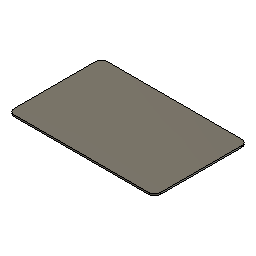
Card 3D File (Autodesk Fusion 360 design; units mm, degrees)
part number: 2026-02-12-13-33-12-488
Autodesk Fusion 360 part; units mm, degrees
(part 1 of 7)
sketch "Sketch1" plane through (0, 0, 0) normal (1, 0, 0) x (0, 0, -1)
  line L0 (-15.175, 11) -> (-93.825, 11)
  line L1 (-97, 14.175) -> (-97, 61.825)
  line L2 (-93.825, 65) -> (-15.175, 65)
  line L3 (-12, 61.825) -> (-12, 14.175)
  arc A0 (-12, 61.825) -> (-15.175, 65) centre (-15.175, 61.825) ccw
  arc A1 (-93.825, 65) -> (-97, 61.825) centre (-93.825, 61.825) ccw
  arc A2 (-97, 14.175) -> (-93.825, 11) centre (-93.825, 14.175) ccw
  arc A3 (-15.175, 11) -> (-12, 14.175) centre (-15.175, 14.175) ccw
  point P0 (-12, 11)
  point P1 (-97, 11)
  point P2 (-12, 65)
  dimension "d1" = 85
  dimension "d2" = 54
  dimension "d3" = 3.175
  dimension "d4" = 3.175
  dimension "d5" = 3.175
  constraint horizontal L0
  constraint vertical L1
  constraint horizontal L2
  constraint vertical L3
  constraint coincident P2 L2
  constraint coincident P2 L3
  constraint tangent L2 A0
  constraint tangent L3 A0
  constraint tangent L1 A1
  constraint tangent L2 A1
  constraint coincident P1 L0
  constraint coincident P1 L1
  constraint tangent L0 A2
  constraint tangent L1 A2
  constraint coincident P0 L0
  constraint coincident P0 L3
  constraint tangent L0 A3
  constraint tangent L3 A3
  constraint equal A2 A3
  measures "d1" distance of P0 P1
  measures "d2" distance of P0 P2
  measures "d3" radius of A0
  measures "d4" radius of A1
  measures "d5" radius of A2
extrude "Extrude1" add sketch "Sketch1" along normal blind 1 makes body 1
move_body "Move1" bodies 1 to x (0, -1, 0) y (1, 0, 0) z (0, 0, 1) at (-11, 11, 0)
move_body "Move2" bodies 1 to x (1, 0, 0) y (0, 1, 0) z (0, 0, 1) at (0, -10, 0)
sketch "Sketch2" plane through (0, 1, 0) normal (0, 1, 0) x (-1, 0, 0)
  arc A0 (0, 93.825) -> (-3.175, 97) centre (-3.175, 93.825) ccw
  line L0 (-3.175, 97) -> (-50.825, 97)
  arc A1 (-50.825, 97) -> (-54, 93.825) centre (-50.825, 93.825) ccw
  line L1 (-54, 93.825) -> (-54, 15.175)
  arc A2 (-54, 15.175) -> (-50.825, 12) centre (-50.825, 15.175) ccw
  line L2 (-50.825, 12) -> (-3.175, 12)
  arc A3 (-3.175, 12) -> (0, 15.175) centre (-3.175, 15.175) ccw
  line L3 (0, 15.175) -> (0, 93.825)
  line L4 (-2.9236, 18.2465) -> (-2.9236, 17.8828)
  line L5 (-2.9236, 17.8828) -> (-5.1949, 18.7001)
  line L6 (-5.1949, 18.7001) -> (-5.1949, 19.096)
  line L7 (-5.1949, 19.096) -> (-2.9236, 19.9134)
  line L8 (-2.9236, 19.9134) -> (-2.9236, 19.5496)
  line L9 (-2.9236, 19.5496) -> (-4.7824, 18.9075)
  line L10 (-4.7824, 18.9075) -> (-4.7824, 18.8898)
  line L11 (-4.7824, 18.8898) -> (-2.9236, 18.2465)
  line L12 (-3.813, 18.3075) -> (-3.813, 19.4875)
  line L13 (-3.813, 19.4875) -> (-3.5248, 19.4875)
  line L14 (-3.5248, 19.4875) -> (-3.5248, 18.3075)
  line L15 (-3.5248, 18.3075) -> (-3.813, 18.3075)
  line L16 (-2.9236, 20.2148) -> (-4.627, 20.2148)
  line L17 (-4.627, 20.2148) -> (-4.627, 20.533)
  line L18 (-4.627, 20.533) -> (-4.3498, 20.533)
  line L19 (-4.3498, 20.533) -> (-4.3498, 20.5541)
  spline S0 degree 3 poles (-4.3498, 20.5541) (-4.4437, 20.5896) (-4.5169, 20.6476) (-4.5694, 20.7282) knots 0 0 0 0 1 1 1 1
  spline S1 degree 3 poles (-4.5694, 20.7282) (-4.6226, 20.8088) (-4.6492, 20.9053) (-4.6492, 21.0177) knots 0 0 0 0 1 1 1 1
  spline S2 degree 3 poles (-4.6492, 21.0177) (-4.6492, 21.1315) (-4.6226, 21.2269) (-4.5694, 21.3038) knots 0 0 0 0 1 1 1 1
  spline S3 degree 3 poles (-4.5694, 21.3038) (-4.5161, 21.3814) (-4.4429, 21.4387) (-4.3498, 21.4757) knots 0 0 0 0 1 1 1 1
  line L20 (-4.3498, 21.4757) -> (-4.3498, 21.4935)
  spline S4 degree 3 poles (-4.3498, 21.4935) (-4.4407, 21.5341) (-4.5132, 21.5988) (-4.5672, 21.6875) knots 0 0 0 0 1 1 1 1
  spline S5 degree 3 poles (-4.5672, 21.6875) (-4.6219, 21.7763) (-4.6492, 21.882) (-4.6492, 22.0047) knots 0 0 0 0 1 1 1 1
  spline S6 degree 3 poles (-4.6492, 22.0047) (-4.6492, 22.1592) (-4.6008, 22.2853) (-4.504, 22.3829) knots 0 0 0 0 1 1 1 1
  spline S7 degree 3 poles (-4.504, 22.3829) (-4.4072, 22.4812) (-4.2612, 22.5304) (-4.066, 22.5304) knots 0 0 0 0 1 1 1 1
  line L21 (-4.066, 22.5304) -> (-2.9236, 22.5304)
  line L22 (-2.9236, 22.5304) -> (-2.9236, 22.1988)
  line L23 (-2.9236, 22.1988) -> (-4.0349, 22.1988)
  spline S8 degree 3 poles (-4.0349, 22.1988) (-4.1501, 22.1988) (-4.2337, 22.1674) (-4.2855, 22.1045) knots 0 0 0 0 1 1 1 1
  spline S9 degree 3 poles (-4.2855, 22.1045) (-4.3372, 22.0417) (-4.3631, 21.9666) (-4.3631, 21.8794) knots 0 0 0 0 1 1 1 1
  spline S10 degree 3 poles (-4.3631, 21.8794) (-4.3631, 21.7714) (-4.3299, 21.6875) (-4.2633, 21.6276) knots 0 0 0 0 1 1 1 1
  spline S11 degree 3 poles (-4.2633, 21.6276) (-4.1974, 21.5677) (-4.1128, 21.5378) (-4.0093, 21.5378) knots 0 0 0 0 1 1 1 1
  line L24 (-4.0093, 21.5378) -> (-2.9236, 21.5378)
  line L25 (-2.9236, 21.5378) -> (-2.9236, 21.2073)
  line L26 (-2.9236, 21.2073) -> (-4.056, 21.2073)
  spline S12 degree 3 poles (-4.056, 21.2073) (-4.1484, 21.2073) (-4.2226, 21.1785) (-4.2788, 21.1208) knots 0 0 0 0 1 1 1 1
  spline S13 degree 3 poles (-4.2788, 21.1208) (-4.335, 21.0632) (-4.3631, 20.9881) (-4.3631, 20.8957) knots 0 0 0 0 1 1 1 1
  spline S14 degree 3 poles (-4.3631, 20.8957) (-4.3631, 20.8328) (-4.3466, 20.7748) (-4.3132, 20.7216) knots 0 0 0 0 1 1 1 1
  spline S15 degree 3 poles (-4.3132, 20.7216) (-4.2807, 20.6691) (-4.2352, 20.6266) (-4.1768, 20.594) knots 0 0 0 0 1 1 1 1
  spline S16 degree 3 poles (-4.1768, 20.594) (-4.1184, 20.5622) (-4.0508, 20.5463) (-3.9738, 20.5463) knots 0 0 0 0 1 1 1 1
  line L27 (-3.9738, 20.5463) -> (-2.9236, 20.5463)
  line L28 (-2.9236, 20.5463) -> (-2.9236, 20.2148)
  line L29 (-2.9236, 22.9748) -> (-4.627, 22.9748)
  line L30 (-4.627, 22.9748) -> (-4.627, 23.2953)
  line L31 (-4.627, 23.2953) -> (-4.3564, 23.2953)
  line L32 (-4.3564, 23.2953) -> (-4.3564, 23.3131)
  spline S17 degree 3 poles (-4.3564, 23.3131) (-4.4482, 23.3441) (-4.5202, 23.3988) (-4.5727, 23.4772) knots 0 0 0 0 1 1 1 1
  spline S18 degree 3 poles (-4.5727, 23.4772) (-4.6259, 23.5563) (-4.6526, 23.6458) (-4.6526, 23.7456) knots 0 0 0 0 1 1 1 1
  spline S19 degree 3 poles (-4.6526, 23.7456) (-4.6526, 23.7663) (-4.6518, 23.7907) (-4.6504, 23.8188) knots 0 0 0 0 1 1 1 1
  spline S20 degree 3 poles (-4.6504, 23.8188) (-4.6489, 23.8476) (-4.647, 23.8702) (-4.6448, 23.8864) knots 0 0 0 0 1 1 1 1
  line L33 (-4.6448, 23.8864) -> (-4.3277, 23.8864)
  spline S21 degree 3 poles (-4.3277, 23.8864) (-4.3313, 23.8731) (-4.3355, 23.8495) (-4.3398, 23.8155) knots 0 0 0 0 1 1 1 1
  spline S22 degree 3 poles (-4.3398, 23.8155) (-4.345, 23.7814) (-4.3477, 23.7474) (-4.3477, 23.7134) knots 0 0 0 0 1 1 1 1
  spline S23 degree 3 poles (-4.3477, 23.7134) (-4.3477, 23.6351) (-4.3309, 23.5652) (-4.2977, 23.5038) knots 0 0 0 0 1 1 1 1
  spline S24 degree 3 poles (-4.2977, 23.5038) (-4.2652, 23.4432) (-4.2198, 23.3951) (-4.1612, 23.3596) knots 0 0 0 0 1 1 1 1
  spline S25 degree 3 poles (-4.1612, 23.3596) (-4.1036, 23.3242) (-4.0379, 23.3064) (-3.9638, 23.3064) knots 0 0 0 0 1 1 1 1
  line L34 (-3.9638, 23.3064) -> (-2.9236, 23.3064)
  line L35 (-2.9236, 23.3064) -> (-2.9236, 22.9748)
  line L36 (-2.9236, 24.1734) -> (-4.627, 24.1734)
  line L37 (-4.627, 24.1734) -> (-4.627, 24.505)
  line L38 (-4.627, 24.505) -> (-2.9236, 24.505)
  line L39 (-2.9236, 24.505) -> (-2.9236, 24.1734)
  spline S26 degree 3 poles (-4.89, 24.3408) (-4.89, 24.2832) (-4.9092, 24.2336) (-4.9476, 24.1922) knots 0 0 0 0 1 1 1 1
  spline S27 degree 3 poles (-4.9476, 24.1922) (-4.9868, 24.1516) (-5.0333, 24.1312) (-5.0873, 24.1312) knots 0 0 0 0 1 1 1 1
  spline S28 degree 3 poles (-5.0873, 24.1312) (-5.142, 24.1312) (-5.1887, 24.1516) (-5.2271, 24.1922) knots 0 0 0 0 1 1 1 1
  spline S29 degree 3 poles (-5.2271, 24.1922) (-5.2663, 24.2336) (-5.2858, 24.2832) (-5.2858, 24.3408) knots 0 0 0 0 1 1 1 1
  spline S30 degree 3 poles (-5.2858, 24.3408) (-5.2858, 24.3985) (-5.2663, 24.4477) (-5.2271, 24.4883) knots 0 0 0 0 1 1 1 1
  spline S31 degree 3 poles (-5.2271, 24.4883) (-5.1887, 24.5297) (-5.142, 24.5504) (-5.0873, 24.5504) knots 0 0 0 0 1 1 1 1
  spline S32 degree 3 poles (-5.0873, 24.5504) (-5.0333, 24.5504) (-4.9868, 24.5297) (-4.9476, 24.4883) knots 0 0 0 0 1 1 1 1
  spline S33 degree 3 poles (-4.9476, 24.4883) (-4.9092, 24.4477) (-4.89, 24.3985) (-4.89, 24.3408) knots 0 0 0 0 1 1 1 1
  line L40 (-4.627, 25.7462) -> (-4.3609, 25.7462)
  line L41 (-4.3609, 25.7462) -> (-4.3609, 24.8158)
  line L42 (-4.3609, 24.8158) -> (-4.627, 24.8158)
  line L43 (-4.627, 24.8158) -> (-4.627, 25.7462)
  line L44 (-5.0352, 25.0653) -> (-5.0352, 25.3969)
  line L45 (-5.0352, 25.3969) -> (-3.4237, 25.3969)
  spline S34 degree 3 poles (-3.4237, 25.3969) (-3.3595, 25.3969) (-3.311, 25.4065) (-3.2785, 25.4257) knots 0 0 0 0 1 1 1 1
  spline S35 degree 3 poles (-3.2785, 25.4257) (-3.2466, 25.445) (-3.2249, 25.4697) (-3.2131, 25.5) knots 0 0 0 0 1 1 1 1
  spline S36 degree 3 poles (-3.2131, 25.5) (-3.202, 25.5311) (-3.1964, 25.5647) (-3.1964, 25.601) knots 0 0 0 0 1 1 1 1
  spline S37 degree 3 poles (-3.1964, 25.601) (-3.1964, 25.6276) (-3.1982, 25.6509) (-3.202, 25.6708) knots 0 0 0 0 1 1 1 1
  spline S38 degree 3 poles (-3.202, 25.6708) (-3.2057, 25.6908) (-3.2087, 25.7063) (-3.2109, 25.7174) knots 0 0 0 0 1 1 1 1
  line L46 (-3.2109, 25.7174) -> (-2.937, 25.7773)
  spline S39 degree 3 poles (-2.937, 25.7773) (-2.9295, 25.7581) (-2.9222, 25.7307) (-2.9147, 25.6952) knots 0 0 0 0 1 1 1 1
  spline S40 degree 3 poles (-2.9147, 25.6952) (-2.9066, 25.6597) (-2.9022, 25.6154) (-2.9014, 25.5621) knots 0 0 0 0 1 1 1 1
  spline S41 degree 3 poles (-2.9014, 25.5621) (-2.9, 25.4749) (-2.9155, 25.3936) (-2.9481, 25.3182) knots 0 0 0 0 1 1 1 1
  spline S42 degree 3 poles (-2.9481, 25.3182) (-2.9806, 25.2427) (-3.0309, 25.1818) (-3.0988, 25.1352) knots 0 0 0 0 1 1 1 1
  spline S43 degree 3 poles (-3.0988, 25.1352) (-3.1669, 25.0886) (-3.2523, 25.0653) (-3.355, 25.0653) knots 0 0 0 0 1 1 1 1
  line L47 (-3.355, 25.0653) -> (-5.0352, 25.0653)
  spline S44 degree 3 poles (-12.1187, 79.4371) (-12.12, 79.1129) (-12.1998, 78.8339) (-12.3581, 78.6001) knots 0 0 0 0 1 1 1 1
  spline S45 degree 3 poles (-12.3581, 78.6001) (-12.5164, 78.3675) (-12.7458, 78.1884) (-13.0463, 78.0628) knots 0 0 0 0 1 1 1 1
  spline S46 degree 3 poles (-13.0463, 78.0628) (-13.3467, 77.9384) (-13.708, 77.8767) (-14.1302, 77.8779) knots 0 0 0 0 1 1 1 1
  spline S47 degree 3 poles (-14.1302, 77.8779) (-14.5514, 77.8779) (-14.9102, 77.9402) (-15.2069, 78.0647) knots 0 0 0 0 1 1 1 1
  spline S48 degree 3 poles (-15.2069, 78.0647) (-15.5034, 78.1904) (-15.7291, 78.3695) (-15.8836, 78.602) knots 0 0 0 0 1 1 1 1
  spline S49 degree 3 poles (-15.8836, 78.602) (-16.0395, 78.8358) (-16.1174, 79.1142) (-16.1174, 79.4371) knots 0 0 0 0 1 1 1 1
  spline S50 degree 3 poles (-16.1174, 79.4371) (-16.1174, 79.7602) (-16.0395, 80.0379) (-15.8836, 80.2704) knots 0 0 0 0 1 1 1 1
  spline S51 degree 3 poles (-15.8836, 80.2704) (-15.7278, 80.5042) (-15.5015, 80.6839) (-15.205, 80.8096) knots 0 0 0 0 1 1 1 1
  spline S52 degree 3 poles (-15.205, 80.8096) (-14.9096, 80.9353) (-14.5514, 80.9976) (-14.1302, 80.9962) knots 0 0 0 0 1 1 1 1
  spline S53 degree 3 poles (-14.1302, 80.9962) (-13.7068, 80.9962) (-13.3448, 80.9335) (-13.0444, 80.8078) knots 0 0 0 0 1 1 1 1
  spline S54 degree 3 poles (-13.0444, 80.8078) (-12.744, 80.6833) (-12.5146, 80.5048) (-12.3562, 80.2723) knots 0 0 0 0 1 1 1 1
  spline S55 degree 3 poles (-12.3562, 80.2723) (-12.1979, 80.0398) (-12.1187, 79.7614) (-12.1187, 79.4371) knots 0 0 0 0 1 1 1 1
  spline S56 degree 3 poles (-12.7955, 79.4371) (-12.7955, 79.6583) (-12.9068, 79.8349) (-13.1292, 79.9669) knots 0 0 0 0 1 1 1 1
  spline S57 degree 3 poles (-13.1292, 79.9669) (-13.3517, 80.0988) (-13.6854, 80.1643) (-14.1302, 80.163) knots 0 0 0 0 1 1 1 1
  spline S58 degree 3 poles (-14.1302, 80.163) (-14.4232, 80.163) (-14.6671, 80.1329) (-14.8618, 80.0725) knots 0 0 0 0 1 1 1 1
  spline S59 degree 3 poles (-14.8618, 80.0725) (-15.0567, 80.0134) (-15.2031, 79.9293) (-15.301, 79.8198) knots 0 0 0 0 1 1 1 1
  spline S60 degree 3 poles (-15.301, 79.8198) (-15.3991, 79.7117) (-15.4481, 79.5842) (-15.4481, 79.4371) knots 0 0 0 0 1 1 1 1
  spline S61 degree 3 poles (-15.4481, 79.4371) (-15.4481, 79.2172) (-15.3382, 79.0412) (-15.1182, 78.9093) knots 0 0 0 0 1 1 1 1
  spline S62 degree 3 poles (-15.1182, 78.9093) (-14.8983, 78.7773) (-14.569, 78.7107) (-14.1302, 78.7094) knots 0 0 0 0 1 1 1 1
  spline S63 degree 3 poles (-14.1302, 78.7094) (-13.8337, 78.7094) (-13.5861, 78.7389) (-13.3874, 78.798) knots 0 0 0 0 1 1 1 1
  spline S64 degree 3 poles (-13.3874, 78.798) (-13.1902, 78.8584) (-13.0419, 78.9432) (-12.9426, 79.0525) knots 0 0 0 0 1 1 1 1
  spline S65 degree 3 poles (-12.9426, 79.0525) (-12.8445, 79.1619) (-12.7955, 79.2901) (-12.7955, 79.4371) knots 0 0 0 0 1 1 1 1
  line L48 (-12.2035, 81.5783) -> (-12.7917, 81.5783)
  line L49 (-12.7917, 81.5783) -> (-14.0643, 82.9528)
  spline S66 degree 3 poles (-14.0643, 82.9528) (-14.1774, 83.0697) (-14.2792, 83.1678) (-14.3698, 83.247) knots 0 0 0 0 1 1 1 1
  spline S67 degree 3 poles (-14.3698, 83.247) (-14.4602, 83.3274) (-14.5489, 83.3883) (-14.6355, 83.4298) knots 0 0 0 0 1 1 1 1
  spline S68 degree 3 poles (-14.6355, 83.4298) (-14.7236, 83.4712) (-14.8184, 83.492) (-14.9202, 83.492) knots 0 0 0 0 1 1 1 1
  spline S69 degree 3 poles (-14.9202, 83.492) (-15.0334, 83.492) (-15.1308, 83.4662) (-15.2125, 83.4147) knots 0 0 0 0 1 1 1 1
  spline S70 degree 3 poles (-15.2125, 83.4147) (-15.2954, 83.3631) (-15.359, 83.2927) (-15.4029, 83.2036) knots 0 0 0 0 1 1 1 1
  spline S71 degree 3 poles (-15.4029, 83.2036) (-15.4481, 83.1142) (-15.4708, 83.0131) (-15.4708, 82.9) knots 0 0 0 0 1 1 1 1
  spline S72 degree 3 poles (-15.4708, 82.9) (-15.4708, 82.7818) (-15.4469, 82.6787) (-15.3991, 82.5908) knots 0 0 0 0 1 1 1 1
  spline S73 degree 3 poles (-15.3991, 82.5908) (-15.3513, 82.5028) (-15.2829, 82.435) (-15.1936, 82.3872) knots 0 0 0 0 1 1 1 1
  spline S74 degree 3 poles (-15.1936, 82.3872) (-15.1045, 82.3394) (-14.9981, 82.3155) (-14.8751, 82.3155) knots 0 0 0 0 1 1 1 1
  line L50 (-14.8751, 82.3155) -> (-14.8751, 81.5407)
  spline S75 degree 3 poles (-14.8751, 81.5407) (-15.1277, 81.5407) (-15.347, 81.5979) (-15.5329, 81.7123) knots 0 0 0 0 1 1 1 1
  spline S76 degree 3 poles (-15.5329, 81.7123) (-15.7191, 81.8266) (-15.8629, 81.9868) (-15.9647, 82.193) knots 0 0 0 0 1 1 1 1
  spline S77 degree 3 poles (-15.9647, 82.193) (-16.0665, 82.3991) (-16.1174, 82.6367) (-16.1174, 82.9056) knots 0 0 0 0 1 1 1 1
  spline S78 degree 3 poles (-16.1174, 82.9056) (-16.1174, 83.1822) (-16.0684, 83.4229) (-15.9705, 83.6278) knots 0 0 0 0 1 1 1 1
  spline S79 degree 3 poles (-15.9705, 83.6278) (-15.8736, 83.8339) (-15.7392, 83.9941) (-15.567, 84.1084) knots 0 0 0 0 1 1 1 1
  spline S80 degree 3 poles (-15.567, 84.1084) (-15.3947, 84.2229) (-15.1974, 84.28) (-14.975, 84.28) knots 0 0 0 0 1 1 1 1
  spline S81 degree 3 poles (-14.975, 84.28) (-14.8292, 84.28) (-14.6852, 84.2512) (-14.5433, 84.1934) knots 0 0 0 0 1 1 1 1
  spline S82 degree 3 poles (-14.5433, 84.1934) (-14.4012, 84.1367) (-14.2434, 84.0357) (-14.07, 83.8898) knots 0 0 0 0 1 1 1 1
  spline S83 degree 3 poles (-14.07, 83.8898) (-13.8977, 83.744) (-13.691, 83.5385) (-13.4497, 83.2733) knots 0 0 0 0 1 1 1 1
  line L51 (-13.4497, 83.2733) -> (-12.8973, 82.7097)
  line L52 (-12.8973, 82.7097) -> (-12.8709, 82.7097)
  line L53 (-12.8709, 82.7097) -> (-12.8709, 84.3309)
  line L54 (-12.8709, 84.3309) -> (-12.2035, 84.3309)
  line L55 (-12.2035, 84.3309) -> (-12.2035, 81.5783)
  line L56 (-16.2456, 86.6117) -> (-11.6228, 85.3675)
  line L57 (-11.6228, 85.3675) -> (-11.6228, 84.6756)
  line L58 (-11.6228, 84.6756) -> (-16.2456, 85.9198)
  line L59 (-16.2456, 85.9198) -> (-16.2456, 86.6117)
  spline S84 degree 3 poles (-12.1507, 88.4183) (-12.1507, 88.1368) (-12.1991, 87.886) (-12.296, 87.6661) knots 0 0 0 0 1 1 1 1
  spline S85 degree 3 poles (-12.296, 87.6661) (-12.3939, 87.4474) (-12.5285, 87.2745) (-12.6993, 87.1476) knots 0 0 0 0 1 1 1 1
  spline S86 degree 3 poles (-12.6993, 87.1476) (-12.8715, 87.022) (-13.0701, 86.9572) (-13.2952, 86.9535) knots 0 0 0 0 1 1 1 1
  line L60 (-13.2952, 86.9535) -> (-13.2952, 87.7754)
  spline S87 degree 3 poles (-13.2952, 87.7754) (-13.2008, 87.7804) (-13.1179, 87.8112) (-13.0463, 87.8679) knots 0 0 0 0 1 1 1 1
  spline S88 degree 3 poles (-13.0463, 87.8679) (-12.9758, 87.9257) (-12.9212, 88.0023) (-12.8823, 88.0979) knots 0 0 0 0 1 1 1 1
  spline S89 degree 3 poles (-12.8823, 88.0979) (-12.8433, 88.1933) (-12.8237, 88.3009) (-12.8237, 88.4202) knots 0 0 0 0 1 1 1 1
  spline S90 degree 3 poles (-12.8237, 88.4202) (-12.8237, 88.5446) (-12.8458, 88.6546) (-12.8898, 88.7501) knots 0 0 0 0 1 1 1 1
  spline S91 degree 3 poles (-12.8898, 88.7501) (-12.9338, 88.8457) (-12.9947, 88.9205) (-13.0726, 88.9745) knots 0 0 0 0 1 1 1 1
  spline S92 degree 3 poles (-13.0726, 88.9745) (-13.1506, 89.0285) (-13.2405, 89.0556) (-13.3423, 89.0556) knots 0 0 0 0 1 1 1 1
  spline S93 degree 3 poles (-13.3423, 89.0556) (-13.4454, 89.0556) (-13.5364, 89.0267) (-13.6156, 88.9689) knots 0 0 0 0 1 1 1 1
  spline S94 degree 3 poles (-13.6156, 88.9689) (-13.696, 88.9124) (-13.7589, 88.8305) (-13.8042, 88.7237) knots 0 0 0 0 1 1 1 1
  spline S95 degree 3 poles (-13.8042, 88.7237) (-13.8493, 88.6182) (-13.872, 88.4925) (-13.872, 88.3466) knots 0 0 0 0 1 1 1 1
  line L61 (-13.872, 88.3466) -> (-13.872, 87.9866)
  line L62 (-13.872, 87.9866) -> (-14.4716, 87.9866)
  line L63 (-14.4716, 87.9866) -> (-14.4716, 88.3466)
  spline S96 degree 3 poles (-14.4716, 88.3466) (-14.4716, 88.4698) (-14.493, 88.5787) (-14.5356, 88.6728) knots 0 0 0 0 1 1 1 1
  spline S97 degree 3 poles (-14.5356, 88.6728) (-14.5784, 88.7684) (-14.6374, 88.8426) (-14.7128, 88.8953) knots 0 0 0 0 1 1 1 1
  spline S98 degree 3 poles (-14.7128, 88.8953) (-14.7895, 88.9481) (-14.8788, 88.9745) (-14.9806, 88.9745) knots 0 0 0 0 1 1 1 1
  spline S99 degree 3 poles (-14.9806, 88.9745) (-15.0774, 88.9745) (-15.1622, 88.9512) (-15.2352, 88.9047) knots 0 0 0 0 1 1 1 1
  spline S100 degree 3 poles (-15.2352, 88.9047) (-15.3093, 88.8596) (-15.3671, 88.7954) (-15.4086, 88.7125) knots 0 0 0 0 1 1 1 1
  spline S101 degree 3 poles (-15.4086, 88.7125) (-15.45, 88.6308) (-15.4708, 88.5353) (-15.4708, 88.426) knots 0 0 0 0 1 1 1 1
  spline S102 degree 3 poles (-15.4708, 88.426) (-15.4708, 88.3152) (-15.4506, 88.2141) (-15.4105, 88.1224) knots 0 0 0 0 1 1 1 1
  spline S103 degree 3 poles (-15.4105, 88.1224) (-15.3715, 88.0306) (-15.3156, 87.957) (-15.2426, 87.9018) knots 0 0 0 0 1 1 1 1
  spline S104 degree 3 poles (-15.2426, 87.9018) (-15.1697, 87.8465) (-15.0843, 87.817) (-14.9862, 87.8132) knots 0 0 0 0 1 1 1 1
  line L64 (-14.9862, 87.8132) -> (-14.9862, 87.0308)
  spline S105 degree 3 poles (-14.9862, 87.0308) (-15.2088, 87.0345) (-15.4047, 87.0981) (-15.5745, 87.2211) knots 0 0 0 0 1 1 1 1
  spline S106 degree 3 poles (-15.5745, 87.2211) (-15.7442, 87.3443) (-15.8768, 87.5103) (-15.9723, 87.7189) knots 0 0 0 0 1 1 1 1
  spline S107 degree 3 poles (-15.9723, 87.7189) (-16.069, 87.9288) (-16.1174, 88.1657) (-16.1174, 88.4297) knots 0 0 0 0 1 1 1 1
  spline S108 degree 3 poles (-16.1174, 88.4297) (-16.1174, 88.6961) (-16.069, 88.9292) (-15.9723, 89.1291) knots 0 0 0 0 1 1 1 1
  spline S109 degree 3 poles (-15.9723, 89.1291) (-15.8755, 89.329) (-15.7448, 89.4842) (-15.5801, 89.5947) knots 0 0 0 0 1 1 1 1
  spline S110 degree 3 poles (-15.5801, 89.5947) (-15.4168, 89.7067) (-15.2333, 89.762) (-15.0297, 89.7607) knots 0 0 0 0 1 1 1 1
  spline S111 degree 3 poles (-15.0297, 89.7607) (-14.8134, 89.762) (-14.633, 89.6947) (-14.4886, 89.559) knots 0 0 0 0 1 1 1 1
  spline S112 degree 3 poles (-14.4886, 89.559) (-14.344, 89.4245) (-14.2522, 89.2492) (-14.2133, 89.0329) knots 0 0 0 0 1 1 1 1
  line L65 (-14.2133, 89.0329) -> (-14.1832, 89.0329)
  spline S113 degree 3 poles (-14.1832, 89.0329) (-14.1466, 89.317) (-14.048, 89.5332) (-13.8871, 89.6816) knots 0 0 0 0 1 1 1 1
  spline S114 degree 3 poles (-13.8871, 89.6816) (-13.7275, 89.8312) (-13.5277, 89.9052) (-13.2875, 89.9039) knots 0 0 0 0 1 1 1 1
  spline S115 degree 3 poles (-13.2875, 89.9039) (-13.0676, 89.9052) (-12.8722, 89.8418) (-12.7013, 89.7136) knots 0 0 0 0 1 1 1 1
  spline S116 degree 3 poles (-12.7013, 89.7136) (-12.5303, 89.5866) (-12.3959, 89.4113) (-12.2978, 89.1875) knots 0 0 0 0 1 1 1 1
  spline S117 degree 3 poles (-12.2978, 89.1875) (-12.1998, 88.9639) (-12.1507, 88.7075) (-12.1507, 88.4183) knots 0 0 0 0 1 1 1 1
  spline S118 degree 3 poles (-12.1187, 92.0047) (-12.12, 91.6804) (-12.1998, 91.4014) (-12.3581, 91.1676) knots 0 0 0 0 1 1 1 1
  spline S119 degree 3 poles (-12.3581, 91.1676) (-12.5164, 90.9351) (-12.7458, 90.756) (-13.0463, 90.6303) knots 0 0 0 0 1 1 1 1
  spline S120 degree 3 poles (-13.0463, 90.6303) (-13.3467, 90.5059) (-13.708, 90.4443) (-14.1302, 90.4456) knots 0 0 0 0 1 1 1 1
  spline S121 degree 3 poles (-14.1302, 90.4456) (-14.5514, 90.4456) (-14.9102, 90.5077) (-15.2069, 90.6322) knots 0 0 0 0 1 1 1 1
  spline S122 degree 3 poles (-15.2069, 90.6322) (-15.5034, 90.7579) (-15.7291, 90.937) (-15.8836, 91.1695) knots 0 0 0 0 1 1 1 1
  spline S123 degree 3 poles (-15.8836, 91.1695) (-16.0395, 91.4033) (-16.1174, 91.6817) (-16.1174, 92.0047) knots 0 0 0 0 1 1 1 1
  spline S124 degree 3 poles (-16.1174, 92.0047) (-16.1174, 92.3277) (-16.0395, 92.6054) (-15.8836, 92.8379) knots 0 0 0 0 1 1 1 1
  spline S125 degree 3 poles (-15.8836, 92.8379) (-15.7278, 93.0719) (-15.5015, 93.2516) (-15.205, 93.3773) knots 0 0 0 0 1 1 1 1
  spline S126 degree 3 poles (-15.205, 93.3773) (-14.9096, 93.5028) (-14.5514, 93.5651) (-14.1302, 93.5639) knots 0 0 0 0 1 1 1 1
  spline S127 degree 3 poles (-14.1302, 93.5639) (-13.7068, 93.5639) (-13.3448, 93.501) (-13.0444, 93.3753) knots 0 0 0 0 1 1 1 1
  spline S128 degree 3 poles (-13.0444, 93.3753) (-12.744, 93.251) (-12.5146, 93.0725) (-12.3562, 92.8398) knots 0 0 0 0 1 1 1 1
  spline S129 degree 3 poles (-12.3562, 92.8398) (-12.1979, 92.6073) (-12.1187, 92.3289) (-12.1187, 92.0047) knots 0 0 0 0 1 1 1 1
  spline S130 degree 3 poles (-12.7955, 92.0047) (-12.7955, 92.2258) (-12.9068, 92.4024) (-13.1292, 92.5346) knots 0 0 0 0 1 1 1 1
  spline S131 degree 3 poles (-13.1292, 92.5346) (-13.3517, 92.6665) (-13.6854, 92.7318) (-14.1302, 92.7305) knots 0 0 0 0 1 1 1 1
  spline S132 degree 3 poles (-14.1302, 92.7305) (-14.4232, 92.7305) (-14.6671, 92.7004) (-14.8618, 92.6401) knots 0 0 0 0 1 1 1 1
  spline S133 degree 3 poles (-14.8618, 92.6401) (-15.0567, 92.5809) (-15.2031, 92.4968) (-15.301, 92.3875) knots 0 0 0 0 1 1 1 1
  spline S134 degree 3 poles (-15.301, 92.3875) (-15.3991, 92.2794) (-15.4481, 92.1518) (-15.4481, 92.0047) knots 0 0 0 0 1 1 1 1
  spline S135 degree 3 poles (-15.4481, 92.0047) (-15.4481, 91.7847) (-15.3382, 91.6087) (-15.1182, 91.4768) knots 0 0 0 0 1 1 1 1
  spline S136 degree 3 poles (-15.1182, 91.4768) (-14.8983, 91.3449) (-14.569, 91.2782) (-14.1302, 91.2769) knots 0 0 0 0 1 1 1 1
  spline S137 degree 3 poles (-14.1302, 91.2769) (-13.8337, 91.2769) (-13.5861, 91.3064) (-13.3874, 91.3656) knots 0 0 0 0 1 1 1 1
  spline S138 degree 3 poles (-13.3874, 91.3656) (-13.1902, 91.4259) (-13.0419, 91.5107) (-12.9426, 91.6201) knots 0 0 0 0 1 1 1 1
  spline S139 degree 3 poles (-12.9426, 91.6201) (-12.8445, 91.7294) (-12.7955, 91.8576) (-12.7955, 92.0047) knots 0 0 0 0 1 1 1 1
  spline S140 degree 3 poles (-48.5277, 92.7546) (-48.5876, 92.8726) (-48.5469, 92.9888) (-48.4658, 93.03) knots 0 0 0 0 1 1 1 1
  line L66 (-48.4658, 93.03) -> (-48.4623, 93.0318)
  line L67 (-48.4623, 93.0318) -> (-48.4588, 93.0338)
  spline S141 degree 3 poles (-48.4588, 93.0338) (-47.5901, 93.5364) (-46.5968, 93.8317) (-45.5192, 93.8373) knots 0 0 0 0 1 1 1 1
  spline S142 degree 3 poles (-45.5192, 93.8373) (-44.4427, 93.8431) (-43.4474, 93.5591) (-42.574, 93.0667) knots 0 0 0 0 1 1 1 1
  spline S143 degree 3 poles (-42.574, 93.0667) (-42.4748, 93.0041) (-42.447, 92.8992) (-42.4965, 92.7928) knots 0 0 0 0 1 1 1 1
  spline S144 degree 3 poles (-42.4965, 92.7928) (-42.5596, 92.696) (-42.6642, 92.6696) (-42.7699, 92.7198) knots 0 0 0 0 1 1 1 1
  spline S145 degree 3 poles (-42.7699, 92.7198) (-43.5795, 93.1942) (-44.5173, 93.4496) (-45.5171, 93.4443) knots 0 0 0 0 1 1 1 1
  spline S146 degree 3 poles (-45.5171, 93.4443) (-46.5195, 93.4389) (-47.4538, 93.151) (-48.2554, 92.6912) knots 0 0 0 0 1 1 1 1
  spline S147 degree 3 poles (-48.2554, 92.6912) (-48.3724, 92.6336) (-48.487, 92.6742) (-48.5277, 92.7546) knots 0 0 0 0 1 1 1 1
  spline S148 degree 3 poles (-47.8872, 91.5327) (-47.9426, 91.6486) (-47.902, 91.7616) (-47.8223, 91.8021) knots 0 0 0 0 1 1 1 1
  line L68 (-47.8223, 91.8021) -> (-47.8171, 91.8047)
  line L69 (-47.8171, 91.8047) -> (-47.8121, 91.8076)
  spline S149 degree 3 poles (-47.8121, 91.8076) (-47.1359, 92.2224) (-46.356, 92.453) (-45.5119, 92.4575) knots 0 0 0 0 1 1 1 1
  spline S150 degree 3 poles (-45.5119, 92.4575) (-44.6681, 92.4619) (-43.8861, 92.24) (-43.2058, 91.8328) knots 0 0 0 0 1 1 1 1
  spline S151 degree 3 poles (-43.2058, 91.8328) (-43.1054, 91.7703) (-43.0771, 91.6649) (-43.1268, 91.5581) knots 0 0 0 0 1 1 1 1
  spline S152 degree 3 poles (-43.1268, 91.5581) (-43.1902, 91.461) (-43.2952, 91.4349) (-43.4012, 91.4856) knots 0 0 0 0 1 1 1 1
  spline S153 degree 3 poles (-43.4012, 91.4856) (-44.0162, 91.8318) (-44.7408, 92.0473) (-45.5097, 92.0431) knots 0 0 0 0 1 1 1 1
  spline S154 degree 3 poles (-45.5097, 92.0431) (-46.2751, 92.039) (-46.9986, 91.8388) (-47.6135, 91.4624) knots 0 0 0 0 1 1 1 1
  spline S155 degree 3 poles (-47.6135, 91.4624) (-47.7185, 91.4115) (-47.8231, 91.4367) (-47.8872, 91.5327) knots 0 0 0 0 1 1 1 1
  spline S156 degree 3 poles (-47.2523, 90.2965) (-47.3004, 90.363) (-47.2833, 90.4878) (-47.1841, 90.5618) knots 0 0 0 0 1 1 1 1
  spline S157 degree 3 poles (-47.1841, 90.5618) (-46.6984, 90.868) (-46.1114, 91.0529) (-45.5044, 91.056) knots 0 0 0 0 1 1 1 1
  spline S158 degree 3 poles (-45.5044, 91.056) (-44.8767, 91.0595) (-44.3087, 90.8809) (-43.8196, 90.5797) knots 0 0 0 0 1 1 1 1
  spline S159 degree 3 poles (-43.8196, 90.5797) (-43.7237, 90.5101) (-43.6969, 90.4034) (-43.7512, 90.3115) knots 0 0 0 0 1 1 1 1
  spline S160 degree 3 poles (-43.7512, 90.3115) (-43.8242, 90.2118) (-43.9486, 90.1936) (-44.0156, 90.2407) knots 0 0 0 0 1 1 1 1
  line L70 (-44.0156, 90.2407) -> (-44.0189, 90.2433)
  line L71 (-44.0189, 90.2433) -> (-44.0224, 90.2456)
  spline S161 degree 3 poles (-44.0224, 90.2456) (-44.4497, 90.5122) (-44.9652, 90.6662) (-45.5023, 90.6633) knots 0 0 0 0 1 1 1 1
  spline S162 degree 3 poles (-45.5023, 90.6633) (-46.0393, 90.6604) (-46.5531, 90.5011) (-46.9775, 90.23) knots 0 0 0 0 1 1 1 1
  spline S163 degree 3 poles (-46.9775, 90.23) (-47.0706, 90.1713) (-47.1808, 90.1977) (-47.2523, 90.2965) knots 0 0 0 0 1 1 1 1
  spline S164 degree 3 poles (-46.6301, 89.0896) (-46.6974, 89.1827) (-46.6763, 89.3029) (-46.6011, 89.3572) knots 0 0 0 0 1 1 1 1
  line L72 (-46.6011, 89.3572) -> (-46.5999, 89.3581)
  line L73 (-46.5999, 89.3581) -> (-46.5985, 89.3593)
  spline S165 degree 3 poles (-46.5985, 89.3593) (-46.4398, 89.4795) (-46.2634, 89.5782) (-46.0905, 89.6372) knots 0 0 0 0 1 1 1 1
  spline S166 degree 3 poles (-46.0905, 89.6372) (-45.8871, 89.6992) (-45.6903, 89.7387) (-45.4974, 89.7398) knots 0 0 0 0 1 1 1 1
  spline S167 degree 3 poles (-45.4974, 89.7398) (-45.2944, 89.741) (-45.1023, 89.7214) (-44.9132, 89.6469) knots 0 0 0 0 1 1 1 1
  spline S168 degree 3 poles (-44.9132, 89.6469) (-44.7072, 89.5658) (-44.5492, 89.4873) (-44.3923, 89.371) knots 0 0 0 0 1 1 1 1
  line L74 (-44.3923, 89.371) -> (-44.3911, 89.3698)
  line L75 (-44.3911, 89.3698) -> (-44.3897, 89.3689)
  spline S169 degree 3 poles (-44.3897, 89.3689) (-44.3139, 89.3154) (-44.2915, 89.1955) (-44.3578, 89.1016) knots 0 0 0 0 1 1 1 1
  spline S170 degree 3 poles (-44.3578, 89.1016) (-44.4108, 89.0267) (-44.5289, 89.004) (-44.6223, 89.0679) knots 0 0 0 0 1 1 1 1
  spline S171 degree 3 poles (-44.6223, 89.0679) (-44.7439, 89.1633) (-44.8861, 89.2326) (-45.0251, 89.2781) knots 0 0 0 0 1 1 1 1
  spline S172 degree 3 poles (-45.0251, 89.2781) (-45.1697, 89.3254) (-45.3341, 89.3476) (-45.4953, 89.3466) knots 0 0 0 0 1 1 1 1
  spline S173 degree 3 poles (-45.4953, 89.3466) (-45.6565, 89.3458) (-45.8207, 89.3219) (-45.9649, 89.2731) knots 0 0 0 0 1 1 1 1
  spline S174 degree 3 poles (-45.9649, 89.2731) (-46.1033, 89.2261) (-46.2447, 89.1553) (-46.3652, 89.0587) knots 0 0 0 0 1 1 1 1
  spline S175 degree 3 poles (-46.3652, 89.0587) (-46.4579, 88.9937) (-46.5763, 89.0151) (-46.6301, 89.0896) knots 0 0 0 0 1 1 1 1
  line L76 (-9.9923, 17.8051) -> (-9.9923, 94.3182)
  spline S176 degree 3 poles (-12.1507, 19.233) (-12.1507, 18.9515) (-12.1991, 18.7007) (-12.296, 18.4808) knots 0 0 0 0 1 1 1 1
  spline S177 degree 3 poles (-12.296, 18.4808) (-12.3939, 18.2621) (-12.5285, 18.0892) (-12.6993, 17.9623) knots 0 0 0 0 1 1 1 1
  spline S178 degree 3 poles (-12.6993, 17.9623) (-12.8715, 17.8366) (-13.0701, 17.7719) (-13.2952, 17.7681) knots 0 0 0 0 1 1 1 1
  line L77 (-13.2952, 17.7681) -> (-13.2952, 18.5901)
  spline S179 degree 3 poles (-13.2952, 18.5901) (-13.2008, 18.5951) (-13.1179, 18.6259) (-13.0463, 18.6825) knots 0 0 0 0 1 1 1 1
  spline S180 degree 3 poles (-13.0463, 18.6825) (-12.9758, 18.7403) (-12.9212, 18.817) (-12.8823, 18.9125) knots 0 0 0 0 1 1 1 1
  spline S181 degree 3 poles (-12.8823, 18.9125) (-12.8433, 19.008) (-12.8237, 19.1155) (-12.8237, 19.2349) knots 0 0 0 0 1 1 1 1
  spline S182 degree 3 poles (-12.8237, 19.2349) (-12.8237, 19.3593) (-12.8458, 19.4693) (-12.8898, 19.5648) knots 0 0 0 0 1 1 1 1
  spline S183 degree 3 poles (-12.8898, 19.5648) (-12.9338, 19.6603) (-12.9947, 19.7351) (-13.0726, 19.7892) knots 0 0 0 0 1 1 1 1
  spline S184 degree 3 poles (-13.0726, 19.7892) (-13.1506, 19.8432) (-13.2405, 19.8702) (-13.3423, 19.8702) knots 0 0 0 0 1 1 1 1
  spline S185 degree 3 poles (-13.3423, 19.8702) (-13.4454, 19.8702) (-13.5364, 19.8413) (-13.6156, 19.7835) knots 0 0 0 0 1 1 1 1
  spline S186 degree 3 poles (-13.6156, 19.7835) (-13.696, 19.727) (-13.7589, 19.6453) (-13.8042, 19.5384) knots 0 0 0 0 1 1 1 1
  spline S187 degree 3 poles (-13.8042, 19.5384) (-13.8493, 19.4328) (-13.872, 19.3072) (-13.872, 19.1614) knots 0 0 0 0 1 1 1 1
  line L78 (-13.872, 19.1614) -> (-13.872, 18.8013)
  line L79 (-13.872, 18.8013) -> (-14.4716, 18.8013)
  line L80 (-14.4716, 18.8013) -> (-14.4716, 19.1614)
  spline S188 degree 3 poles (-14.4716, 19.1614) (-14.4716, 19.2845) (-14.493, 19.3933) (-14.5356, 19.4875) knots 0 0 0 0 1 1 1 1
  spline S189 degree 3 poles (-14.5356, 19.4875) (-14.5784, 19.583) (-14.6374, 19.6572) (-14.7128, 19.71) knots 0 0 0 0 1 1 1 1
  spline S190 degree 3 poles (-14.7128, 19.71) (-14.7895, 19.7628) (-14.8788, 19.7892) (-14.9806, 19.7892) knots 0 0 0 0 1 1 1 1
  spline S191 degree 3 poles (-14.9806, 19.7892) (-15.0774, 19.7892) (-15.1622, 19.7659) (-15.2352, 19.7194) knots 0 0 0 0 1 1 1 1
  spline S192 degree 3 poles (-15.2352, 19.7194) (-15.3093, 19.6742) (-15.3671, 19.6101) (-15.4086, 19.5271) knots 0 0 0 0 1 1 1 1
  spline S193 degree 3 poles (-15.4086, 19.5271) (-15.45, 19.4454) (-15.4708, 19.3499) (-15.4708, 19.2405) knots 0 0 0 0 1 1 1 1
  spline S194 degree 3 poles (-15.4708, 19.2405) (-15.4708, 19.1299) (-15.4506, 19.0288) (-15.4105, 18.937) knots 0 0 0 0 1 1 1 1
  spline S195 degree 3 poles (-15.4105, 18.937) (-15.3715, 18.8453) (-15.3156, 18.7717) (-15.2426, 18.7164) knots 0 0 0 0 1 1 1 1
  spline S196 degree 3 poles (-15.2426, 18.7164) (-15.1697, 18.6611) (-15.0843, 18.6316) (-14.9862, 18.6278) knots 0 0 0 0 1 1 1 1
  line L81 (-14.9862, 18.6278) -> (-14.9862, 17.8454)
  spline S197 degree 3 poles (-14.9862, 17.8454) (-15.2088, 17.8492) (-15.4047, 17.9126) (-15.5745, 18.0358) knots 0 0 0 0 1 1 1 1
  spline S198 degree 3 poles (-15.5745, 18.0358) (-15.7442, 18.159) (-15.8768, 18.3249) (-15.9723, 18.5335) knots 0 0 0 0 1 1 1 1
  spline S199 degree 3 poles (-15.9723, 18.5335) (-16.069, 18.7434) (-16.1174, 18.9804) (-16.1174, 19.2443) knots 0 0 0 0 1 1 1 1
  spline S200 degree 3 poles (-16.1174, 19.2443) (-16.1174, 19.5108) (-16.069, 19.7439) (-15.9723, 19.9438) knots 0 0 0 0 1 1 1 1
  spline S201 degree 3 poles (-15.9723, 19.9438) (-15.8755, 20.1436) (-15.7448, 20.2988) (-15.5801, 20.4094) knots 0 0 0 0 1 1 1 1
  spline S202 degree 3 poles (-15.5801, 20.4094) (-15.4168, 20.5213) (-15.2333, 20.5766) (-15.0297, 20.5754) knots 0 0 0 0 1 1 1 1
  spline S203 degree 3 poles (-15.0297, 20.5754) (-14.8134, 20.5766) (-14.633, 20.5094) (-14.4886, 20.3736) knots 0 0 0 0 1 1 1 1
  spline S204 degree 3 poles (-14.4886, 20.3736) (-14.344, 20.2391) (-14.2522, 20.0638) (-14.2133, 19.8476) knots 0 0 0 0 1 1 1 1
  line L82 (-14.2133, 19.8476) -> (-14.1832, 19.8476)
  spline S205 degree 3 poles (-14.1832, 19.8476) (-14.1466, 20.1317) (-14.048, 20.3479) (-13.8871, 20.4962) knots 0 0 0 0 1 1 1 1
  spline S206 degree 3 poles (-13.8871, 20.4962) (-13.7275, 20.6457) (-13.5277, 20.7199) (-13.2875, 20.7186) knots 0 0 0 0 1 1 1 1
  spline S207 degree 3 poles (-13.2875, 20.7186) (-13.0676, 20.7199) (-12.8722, 20.6564) (-12.7013, 20.5282) knots 0 0 0 0 1 1 1 1
  spline S208 degree 3 poles (-12.7013, 20.5282) (-12.5303, 20.4013) (-12.3959, 20.2259) (-12.2978, 20.0022) knots 0 0 0 0 1 1 1 1
  spline S209 degree 3 poles (-12.2978, 20.0022) (-12.1998, 19.7785) (-12.1507, 19.5221) (-12.1507, 19.233) knots 0 0 0 0 1 1 1 1
  spline S210 degree 3 poles (-12.1507, 22.928) (-12.1507, 22.6616) (-12.1998, 22.424) (-12.2978, 22.2154) knots 0 0 0 0 1 1 1 1
  spline S211 degree 3 poles (-12.2978, 22.2154) (-12.3959, 22.008) (-12.531, 21.8433) (-12.7032, 21.7214) knots 0 0 0 0 1 1 1 1
  spline S212 degree 3 poles (-12.7032, 21.7214) (-12.8753, 21.5995) (-13.0726, 21.536) (-13.2952, 21.531) knots 0 0 0 0 1 1 1 1
  line L83 (-13.2952, 21.531) -> (-13.2952, 22.3228)
  spline S213 degree 3 poles (-13.2952, 22.3228) (-13.1456, 22.3316) (-13.0242, 22.3945) (-12.9313, 22.5114) knots 0 0 0 0 1 1 1 1
  spline S214 degree 3 poles (-12.9313, 22.5114) (-12.8383, 22.6283) (-12.7917, 22.7671) (-12.7917, 22.928) knots 0 0 0 0 1 1 1 1
  spline S215 degree 3 poles (-12.7917, 22.928) (-12.7917, 23.0562) (-12.82, 23.1694) (-12.8765, 23.2674) knots 0 0 0 0 1 1 1 1
  spline S216 degree 3 poles (-12.8765, 23.2674) (-12.9345, 23.3667) (-13.0142, 23.444) (-13.1161, 23.4993) knots 0 0 0 0 1 1 1 1
  spline S217 degree 3 poles (-13.1161, 23.4993) (-13.2191, 23.5558) (-13.3372, 23.5841) (-13.4705, 23.5841) knots 0 0 0 0 1 1 1 1
  spline S218 degree 3 poles (-13.4705, 23.5841) (-13.6062, 23.5841) (-13.7257, 23.5552) (-13.8287, 23.4974) knots 0 0 0 0 1 1 1 1
  spline S219 degree 3 poles (-13.8287, 23.4974) (-13.9318, 23.4408) (-14.0122, 23.3623) (-14.07, 23.2617) knots 0 0 0 0 1 1 1 1
  spline S220 degree 3 poles (-14.07, 23.2617) (-14.1277, 23.1612) (-14.1574, 23.0462) (-14.1587, 22.9167) knots 0 0 0 0 1 1 1 1
  spline S221 degree 3 poles (-14.1587, 22.9167) (-14.1587, 22.8036) (-14.1354, 22.6936) (-14.0889, 22.5868) knots 0 0 0 0 1 1 1 1
  spline S222 degree 3 poles (-14.0889, 22.5868) (-14.0423, 22.4812) (-13.9789, 22.3989) (-13.8984, 22.3398) knots 0 0 0 0 1 1 1 1
  line L84 (-13.8984, 22.3398) -> (-14.0286, 21.614)
  line L85 (-14.0286, 21.614) -> (-16.0646, 21.7968)
  line L86 (-16.0646, 21.7968) -> (-16.0646, 24.1573)
  line L87 (-16.0646, 24.1573) -> (-15.3972, 24.1573)
  line L88 (-15.3972, 24.1573) -> (-15.3972, 22.4699)
  line L89 (-15.3972, 22.4699) -> (-14.43, 22.37)
  line L90 (-14.43, 22.37) -> (-14.43, 22.3926)
  spline S223 degree 3 poles (-14.43, 22.3926) (-14.5256, 22.4605) (-14.6048, 22.5629) (-14.6677, 22.6999) knots 0 0 0 0 1 1 1 1
  spline S224 degree 3 poles (-14.6677, 22.6999) (-14.7305, 22.8369) (-14.7619, 22.9903) (-14.7619, 23.1599) knots 0 0 0 0 1 1 1 1
  spline S225 degree 3 poles (-14.7619, 23.1599) (-14.7619, 23.3924) (-14.7072, 23.5998) (-14.5979, 23.7821) knots 0 0 0 0 1 1 1 1
  spline S226 degree 3 poles (-14.5979, 23.7821) (-14.4886, 23.9643) (-14.3384, 24.1082) (-14.1473, 24.2138) knots 0 0 0 0 1 1 1 1
  spline S227 degree 3 poles (-14.1473, 24.2138) (-13.9575, 24.3194) (-13.7388, 24.3716) (-13.4911, 24.3703) knots 0 0 0 0 1 1 1 1
  spline S228 degree 3 poles (-13.4911, 24.3703) (-13.231, 24.3716) (-12.9997, 24.3112) (-12.7974, 24.1893) knots 0 0 0 0 1 1 1 1
  spline S229 degree 3 poles (-12.7974, 24.1893) (-12.5962, 24.0686) (-12.4379, 23.8996) (-12.3223, 23.6822) knots 0 0 0 0 1 1 1 1
  spline S230 degree 3 poles (-12.3223, 23.6822) (-12.2079, 23.466) (-12.1507, 23.2146) (-12.1507, 22.928) knots 0 0 0 0 1 1 1 1
  spline S231 degree 3 poles (-12.1187, 26.6659) (-12.12, 26.3417) (-12.1998, 26.0626) (-12.3581, 25.8289) knots 0 0 0 0 1 1 1 1
  spline S232 degree 3 poles (-12.3581, 25.8289) (-12.5164, 25.5963) (-12.7458, 25.4172) (-13.0463, 25.2915) knots 0 0 0 0 1 1 1 1
  spline S233 degree 3 poles (-13.0463, 25.2915) (-13.3467, 25.1671) (-13.708, 25.1055) (-14.1302, 25.1068) knots 0 0 0 0 1 1 1 1
  spline S234 degree 3 poles (-14.1302, 25.1068) (-14.5514, 25.1068) (-14.9102, 25.169) (-15.2069, 25.2934) knots 0 0 0 0 1 1 1 1
  spline S235 degree 3 poles (-15.2069, 25.2934) (-15.5034, 25.4191) (-15.7291, 25.5982) (-15.8836, 25.8307) knots 0 0 0 0 1 1 1 1
  spline S236 degree 3 poles (-15.8836, 25.8307) (-16.0395, 26.0645) (-16.1174, 26.3429) (-16.1174, 26.6659) knots 0 0 0 0 1 1 1 1
  spline S237 degree 3 poles (-16.1174, 26.6659) (-16.1174, 26.989) (-16.0395, 27.2667) (-15.8836, 27.4993) knots 0 0 0 0 1 1 1 1
  spline S238 degree 3 poles (-15.8836, 27.4993) (-15.7278, 27.733) (-15.5015, 27.9128) (-15.205, 28.0385) knots 0 0 0 0 1 1 1 1
  spline S239 degree 3 poles (-15.205, 28.0385) (-14.9096, 28.1641) (-14.5514, 28.2264) (-14.1302, 28.2251) knots 0 0 0 0 1 1 1 1
  spline S240 degree 3 poles (-14.1302, 28.2251) (-13.7068, 28.2251) (-13.3448, 28.1623) (-13.0444, 28.0366) knots 0 0 0 0 1 1 1 1
  spline S241 degree 3 poles (-13.0444, 28.0366) (-12.744, 27.9122) (-12.5146, 27.7337) (-12.3562, 27.5011) knots 0 0 0 0 1 1 1 1
  spline S242 degree 3 poles (-12.3562, 27.5011) (-12.1979, 27.2686) (-12.1187, 26.9902) (-12.1187, 26.6659) knots 0 0 0 0 1 1 1 1
  spline S243 degree 3 poles (-12.7955, 26.6659) (-12.7955, 26.8872) (-12.9068, 27.0637) (-13.1292, 27.1957) knots 0 0 0 0 1 1 1 1
  spline S244 degree 3 poles (-13.1292, 27.1957) (-13.3517, 27.3277) (-13.6854, 27.393) (-14.1302, 27.3918) knots 0 0 0 0 1 1 1 1
  spline S245 degree 3 poles (-14.1302, 27.3918) (-14.4232, 27.3918) (-14.6671, 27.3616) (-14.8618, 27.3013) knots 0 0 0 0 1 1 1 1
  spline S246 degree 3 poles (-14.8618, 27.3013) (-15.0567, 27.2422) (-15.2031, 27.158) (-15.301, 27.0487) knots 0 0 0 0 1 1 1 1
  spline S247 degree 3 poles (-15.301, 27.0487) (-15.3991, 26.9406) (-15.4481, 26.813) (-15.4481, 26.6659) knots 0 0 0 0 1 1 1 1
  spline S248 degree 3 poles (-15.4481, 26.6659) (-15.4481, 26.446) (-15.3382, 26.27) (-15.1182, 26.1381) knots 0 0 0 0 1 1 1 1
  spline S249 degree 3 poles (-15.1182, 26.1381) (-14.8983, 26.0061) (-14.569, 25.9395) (-14.1302, 25.9382) knots 0 0 0 0 1 1 1 1
  spline S250 degree 3 poles (-14.1302, 25.9382) (-13.8337, 25.9382) (-13.5861, 25.9678) (-13.3874, 26.0268) knots 0 0 0 0 1 1 1 1
  spline S251 degree 3 poles (-13.3874, 26.0268) (-13.1902, 26.0872) (-13.0419, 26.172) (-12.9426, 26.2813) knots 0 0 0 0 1 1 1 1
  spline S252 degree 3 poles (-12.9426, 26.2813) (-12.8445, 26.3907) (-12.7955, 26.5189) (-12.7955, 26.6659) knots 0 0 0 0 1 1 1 1
  line L91 (-12.2035, 29.0686) -> (-15.3708, 30.6692)
  line L92 (-15.3708, 30.6692) -> (-15.3972, 30.6692)
  line L93 (-15.3972, 30.6692) -> (-15.3972, 28.8046)
  line L94 (-15.3972, 28.8046) -> (-16.0646, 28.8046)
  line L95 (-16.0646, 28.8046) -> (-16.0646, 31.5139)
  line L96 (-16.0646, 31.5139) -> (-15.3879, 31.5139)
  line L97 (-15.3879, 31.5139) -> (-12.2035, 29.9113)
  line L98 (-12.2035, 29.9113) -> (-12.2035, 29.0686)
  line L99 (-43.6308, 72.6991) -> (-47.4172, 73.3445)
  line L100 (-47.4172, 73.3445) -> (-47.4172, 74.3764)
  line L101 (-47.4172, 74.3764) -> (-43.6308, 73.7309)
  line L102 (-43.6308, 73.7309) -> (-43.6308, 72.6991)
  spline S253 degree 3 poles (-47.3342, 77.4546) (-47.4414, 77.1585) (-47.4953, 76.8456) (-47.4932, 76.5307) knots 0 0 0 0 1 1 1 1
  spline S254 degree 3 poles (-47.4932, 76.5307) (-47.4932, 75.5123) (-46.9803, 74.7948) (-46.245, 74.7885) knots 0 0 0 0 1 1 1 1
  spline S255 degree 3 poles (-46.245, 74.7885) (-45.7016, 74.7828) (-45.3985, 75.3008) (-45.2176, 75.6918) knots 0 0 0 0 1 1 1 1
  spline S256 degree 3 poles (-45.2176, 75.6918) (-45.0322, 76.0931) (-44.914, 76.2279) (-44.7484, 76.226) knots 0 0 0 0 1 1 1 1
  spline S257 degree 3 poles (-44.7484, 76.226) (-44.495, 76.2234) (-44.3792, 75.9056) (-44.3792, 75.6094) knots 0 0 0 0 1 1 1 1
  spline S258 degree 3 poles (-44.3792, 75.6094) (-44.3792, 75.1967) (-44.4372, 74.9776) (-44.5776, 74.6391) knots 0 0 0 0 1 1 1 1
  line L103 (-44.5776, 74.6391) -> (-44.6377, 74.5064)
  line L104 (-44.6377, 74.5064) -> (-43.7912, 74.3616)
  spline S259 degree 3 poles (-43.7912, 74.3616) (-43.6857, 74.6024) (-43.5941, 75.0476) (-43.5895, 75.5098) knots 0 0 0 0 1 1 1 1
  spline S260 degree 3 poles (-43.5895, 75.5098) (-43.5895, 76.5933) (-44.0964, 77.2966) (-44.8815, 77.3047) knots 0 0 0 0 1 1 1 1
  spline S261 degree 3 poles (-44.8815, 77.3047) (-45.3117, 77.3086) (-45.6392, 77.0343) (-45.9091, 76.4393) knots 0 0 0 0 1 1 1 1
  spline S262 degree 3 poles (-45.9091, 76.4393) (-46.0829, 76.0791) (-46.2008, 75.8585) (-46.3779, 75.8608) knots 0 0 0 0 1 1 1 1
  spline S263 degree 3 poles (-46.3779, 75.8608) (-46.535, 75.8608) (-46.703, 76.0476) (-46.703, 76.451) knots 0 0 0 0 1 1 1 1
  spline S264 degree 3 poles (-46.703, 76.451) (-46.7089, 76.7156) (-46.6596, 76.9782) (-46.5581, 77.2224) knots 0 0 0 0 1 1 1 1
  line L105 (-46.5581, 77.2224) -> (-46.5145, 77.3149)
  line L106 (-46.5145, 77.3149) -> (-47.3342, 77.4546)
  line L107 (-47.4172, 80.1059) -> (-47.4172, 79.312)
  spline S265 degree 3 poles (-47.4172, 79.312) (-47.4172, 79.0661) (-47.35, 78.882) (-47.1047, 78.7739) knots 0 0 0 0 1 1 1 1
  line L108 (-47.1047, 78.7739) -> (-43.6502, 77.2477)
  line L109 (-43.6502, 77.2477) -> (-43.6502, 78.334)
  spline S266 degree 2 poles (-43.6502, 78.334) (-44.1095, 78.508) (-44.2104, 78.548) knots 0 0 0 1 1 1
  line L110 (-44.2104, 78.548) -> (-44.2088, 79.8495)
  spline S267 degree 2 poles (-44.2088, 79.8495) (-44.0782, 79.8798) (-43.6501, 79.973) knots 0 0 0 1 1 1
  line L111 (-43.6501, 79.973) -> (-43.6501, 80.9374)
  line L112 (-43.6501, 80.9374) -> (-47.4172, 80.1059)
  spline S268 degree 2 poles (-44.9831, 78.8436) (-45.201, 78.9287) (-46.0402, 79.2542) knots 0 0 0 1 1 1
  spline S269 degree 3 poles (-46.0402, 79.2542) (-46.0302, 79.248) (-46.2593, 79.3389) (-46.4013, 79.3907) knots 0 0 0 0 1 1 1 1
  line L113 (-46.4013, 79.3907) -> (-46.0752, 79.4605)
  spline S270 degree 2 poles (-46.0752, 79.4605) (-45.1724, 79.6579) (-44.9831, 79.6991) knots 0 0 0 1 1 1
  line L114 (-44.9831, 79.6991) -> (-44.9831, 78.8436)
  line L115 (-47.4172, 71.8234) -> (-44.8442, 70.8166)
  line L116 (-44.8442, 70.8166) -> (-45.3672, 70.7093)
  spline S271 degree 3 poles (-45.3672, 70.7093) (-45.9699, 70.5219) (-46.6229, 69.9379) (-46.9497, 69.2849) knots 0 0 0 0 1 1 1 1
  line L117 (-46.9497, 69.2849) -> (-43.6502, 70.2057)
  line L118 (-43.6502, 70.2057) -> (-43.6513, 71.2937)
  line L119 (-43.6513, 71.2937) -> (-47.4172, 72.9127)
  line L120 (-47.4172, 72.9127) -> (-47.4172, 71.8184)
  line L121 (-47.4173, 69.8316) -> (-47.4173, 68.1765)
  line L122 (-47.4173, 68.1765) -> (-47.3386, 68.1633)
  spline S272 degree 3 poles (-47.3386, 68.1633) (-47.0255, 69.4564) (-46.269, 70.3121) (-45.3603, 70.6673) knots 0 0 0 0 1 1 1 1
  line L123 (-45.3603, 70.6673) -> (-47.0989, 70.3058)
  spline S273 degree 3 poles (-47.0989, 70.3058) (-47.3383, 70.2435) (-47.4097, 70.0627) (-47.418, 69.8388) knots 0 0 0 0 1 1 1 1
  line L124 (-43.5929, 61.4314) -> (-43.5929, 61.0782)
  line L125 (-43.5929, 61.0782) -> (-45.0251, 61.0782)
  line L126 (-45.0251, 61.0782) -> (-45.0251, 61.8889)
  spline S274 degree 3 poles (-45.0251, 61.8889) (-45.0271, 61.9122) (-45.0285, 61.9389) (-45.0285, 61.9663) knots 0 0 0 0 1 1 1 1
  spline S275 degree 3 poles (-45.0285, 61.9663) (-45.0285, 62.0913) (-45.0025, 62.2099) (-44.9554, 62.3169) knots 0 0 0 0 1 1 1 1
  line L127 (-44.9554, 62.3169) -> (-44.9575, 62.3112)
  spline S276 degree 3 poles (-44.9575, 62.3112) (-44.8993, 62.4199) (-44.7884, 62.4925) (-44.6612, 62.4925) knots 0 0 0 0 1 1 1 1
  spline S277 degree 3 poles (-44.6612, 62.4925) (-44.6534, 62.4925) (-44.646, 62.4919) (-44.6386, 62.4916) knots 0 0 0 0 1 1 1 1
  line L128 (-44.6386, 62.4916) -> (-44.6396, 62.4916)
  spline S278 degree 3 poles (-44.6396, 62.4916) (-44.6358, 62.4916) (-44.6311, 62.4919) (-44.6267, 62.4919) knots 0 0 0 0 1 1 1 1
  spline S279 degree 3 poles (-44.6267, 62.4919) (-44.4624, 62.4919) (-44.321, 62.3903) (-44.2594, 62.2444) knots 0 0 0 0 1 1 1 1
  line L129 (-44.2594, 62.2444) -> (-44.2584, 62.2418)
  spline S280 degree 3 poles (-44.2584, 62.2418) (-44.2341, 62.3114) (-44.1925, 62.3698) (-44.1387, 62.4133) knots 0 0 0 0 1 1 1 1
  spline S281 degree 3 poles (-44.1387, 62.4133) (-44.0768, 62.4521) (-44.0024, 62.4749) (-43.9233, 62.4749) knots 0 0 0 0 1 1 1 1
  spline S282 degree 3 poles (-43.9233, 62.4749) (-43.9067, 62.4749) (-43.8908, 62.474) (-43.8746, 62.4723) knots 0 0 0 0 1 1 1 1
  line L130 (-43.8746, 62.4723) -> (-43.8766, 62.4726)
  line L131 (-43.8766, 62.4726) -> (-43.5932, 62.4726)
  line L132 (-43.5932, 62.4726) -> (-43.5932, 62.1198)
  line L133 (-43.5932, 62.1198) -> (-43.7724, 62.1198)
  spline S283 degree 3 poles (-43.7724, 62.1198) (-43.7924, 62.1234) (-43.8157, 62.1255) (-43.8394, 62.1255) knots 0 0 0 0 1 1 1 1
  spline S284 degree 3 poles (-43.8394, 62.1255) (-43.9182, 62.1255) (-43.9919, 62.1025) (-44.0545, 62.0633) knots 0 0 0 0 1 1 1 1
  line L134 (-44.0545, 62.0633) -> (-44.0528, 62.0645)
  spline S285 degree 3 poles (-44.0528, 62.0645) (-44.0947, 62.008) (-44.1201, 61.936) (-44.1201, 61.8582) knots 0 0 0 0 1 1 1 1
  spline S286 degree 3 poles (-44.1201, 61.8582) (-44.1201, 61.8403) (-44.1187, 61.8221) (-44.116, 61.8048) knots 0 0 0 0 1 1 1 1
  line L135 (-44.116, 61.8048) -> (-44.1163, 61.8068)
  line L136 (-44.1163, 61.8068) -> (-44.1163, 61.4313)
  line L137 (-44.1163, 61.4313) -> (-43.5929, 61.4314)
  line L138 (-44.7292, 61.4314) -> (-44.4076, 61.4314)
  line L139 (-44.4076, 61.4314) -> (-44.4076, 61.8583)
  spline S287 degree 3 poles (-44.4076, 61.8583) (-44.4066, 61.8677) (-44.4062, 61.8781) (-44.4062, 61.8892) knots 0 0 0 0 1 1 1 1
  spline S288 degree 3 poles (-44.4062, 61.8892) (-44.4062, 61.941) (-44.4177, 61.9902) (-44.438, 62.0339) knots 0 0 0 0 1 1 1 1
  line L140 (-44.438, 62.0339) -> (-44.437, 62.0319)
  spline S289 degree 3 poles (-44.437, 62.0319) (-44.4651, 62.0759) (-44.5128, 62.1048) (-44.5672, 62.1048) knots 0 0 0 0 1 1 1 1
  spline S290 degree 3 poles (-44.5672, 62.1048) (-44.5699, 62.1048) (-44.5723, 62.1048) (-44.575, 62.1043) knots 0 0 0 0 1 1 1 1
  spline S291 degree 3 poles (-44.575, 62.1043) (-44.5777, 62.1048) (-44.5804, 62.1048) (-44.5834, 62.1048) knots 0 0 0 0 1 1 1 1
  spline S292 degree 3 poles (-44.5834, 62.1048) (-44.6348, 62.1048) (-44.6798, 62.0756) (-44.7031, 62.0326) knots 0 0 0 0 1 1 1 1
  spline S293 degree 3 poles (-44.7031, 62.0326) (-44.7214, 61.9914) (-44.7319, 61.9442) (-44.7319, 61.8941) knots 0 0 0 0 1 1 1 1
  spline S294 degree 3 poles (-44.7319, 61.8941) (-44.7319, 61.884) (-44.7316, 61.8741) (-44.7306, 61.864) knots 0 0 0 0 1 1 1 1
  line L141 (-44.7306, 61.864) -> (-44.7306, 61.8654)
  line L142 (-44.7306, 61.8654) -> (-44.7292, 61.4314)
  line L143 (-43.5932, 58.2989) -> (-43.5932, 56.908)
  line L144 (-43.5932, 56.908) -> (-45.0251, 56.908)
  line L145 (-45.0251, 56.908) -> (-45.0251, 58.3207)
  line L146 (-45.0251, 58.3207) -> (-44.5557, 58.7529)
  line L147 (-44.5557, 58.7529) -> (-45.0251, 59.1997)
  line L148 (-45.0251, 59.1997) -> (-45.0251, 60.3218)
  spline S295 degree 3 poles (-45.0251, 60.3218) (-45.0251, 60.7203) (-44.8706, 60.9139) (-44.5533, 60.9139) knots 0 0 0 0 1 1 1 1
  spline S296 degree 3 poles (-44.5533, 60.9139) (-44.2304, 60.9139) (-44.0734, 60.7137) (-44.0734, 60.303) knots 0 0 0 0 1 1 1 1
  line L149 (-44.0734, 60.303) -> (-44.0734, 59.8639)
  line L150 (-44.0734, 59.8639) -> (-43.5935, 59.8639)
  line L151 (-43.5935, 59.8639) -> (-43.5935, 59.1812)
  line L152 (-43.5935, 59.1812) -> (-44.0667, 58.7487)
  line L153 (-44.0667, 58.7487) -> (-43.5932, 58.2989)
  line L154 (-44.8716, 59.514) -> (-44.3068, 58.9747)
  line L155 (-44.3068, 58.9747) -> (-43.7237, 59.514)
  line L156 (-43.7237, 59.514) -> (-44.8716, 59.514)
  line L157 (-44.1766, 57.2583) -> (-43.8918, 57.2583)
  line L158 (-43.8918, 57.2583) -> (-43.8918, 58.1219)
  line L159 (-43.8918, 58.1219) -> (-44.3119, 58.5211)
  line L160 (-44.3119, 58.5211) -> (-44.7292, 58.1371)
  line L161 (-44.7292, 58.1371) -> (-44.7292, 57.258)
  line L162 (-44.7292, 57.258) -> (-44.4688, 57.258)
  line L163 (-44.4688, 57.258) -> (-44.4688, 58.0292)
  line L164 (-44.4688, 58.0292) -> (-44.1769, 58.0292)
  line L165 (-44.1769, 58.0292) -> (-44.1766, 57.2583)
  line L166 (-44.7288, 59.8639) -> (-44.3643, 59.8639)
  line L167 (-44.3643, 59.8639) -> (-44.3643, 60.3176)
  spline S297 degree 3 poles (-44.3643, 60.3176) (-44.3643, 60.4564) (-44.4333, 60.5363) (-44.5537, 60.5363) knots 0 0 0 0 1 1 1 1
  spline S298 degree 3 poles (-44.5537, 60.5363) (-44.6687, 60.5363) (-44.7292, 60.462) (-44.7292, 60.3215) knots 0 0 0 0 1 1 1 1
  line L168 (-44.7292, 60.3215) -> (-44.7288, 59.8639)
  line L169 (-43.5925, 66.1249) -> (-43.5925, 65.4466)
  line L170 (-43.5925, 65.4466) -> (-43.9003, 65.4466)
  line L171 (-43.9003, 65.4466) -> (-43.9003, 66.1221)
  spline S299 degree 3 poles (-43.9003, 66.1221) (-43.8993, 66.1301) (-43.8986, 66.1391) (-43.8986, 66.1485) knots 0 0 0 0 1 1 1 1